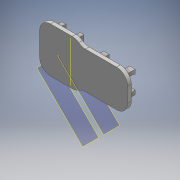
# Autodesk Inventor part: torped2.0
Saved by Autodesk Inventor 2016 (Build 200138000, 138)
## iProperties
Created: 2015-08-25
Part Number: torped2.0
Material: Generic
Document SubType Name: Modeling
Designer: Startic
Density: 1 g/cm^3
Appearance: Default
Author: Startic
Autodesk Inventor part; units mm, degrees
ref_plane "YZ Plane" through (0, 0, 0) normal (1, 0, 0) x (0, 1, 0)
ref_plane "XZ Plane" through (0, 0, 0) normal (0, 1, 0) x (-1, 0, 0)
ref_plane "XY Plane" through (0, 0, 0) normal (0, 0, 1) x (1, 0, 0)
sketch "Sketch1" plane through (0, 0, 0) normal (0, 1, 0) x (-1, 0, 0)
  line L0 (14, 0) -> (-14, 0) projected
  line L1 (0, -17.5) -> (0, 17.5) projected
  line L2 (10, 12.5) -> (-10, 12.5)
  line L3 (-10, 12.5) -> (-10, -12.5)
  line L4 (-10, -12.5) -> (10, -12.5)
  line L5 (10, -12.5) -> (10, 12.5)
  dimension "d0" = 25
  dimension "d1" = 20
  constraints: 8 end point, 2 parallel, 2 symmetric about line, 1 horizontal, 1 perpendicular
  measures "d0" distance of L4.end L2.start
  measures "d1" distance of L3.end L4.end
extrude "Extrusion1" add sketch "Sketch1" along normal blind 2
sketch "Sketch2" plane through (0, 2, 0) normal (0, 1, 0) x (1, 0, 0)
  line L0 (-10, -12.5) -> (10, -12.5) projected
  line L1 (10, -12.5) -> (10, 12.5) projected
  line L2 (10, 12.5) -> (-10, 12.5) projected
  line L3 (-10, 12.5) -> (-10, -12.5) projected
  line L4 (-14, 0) -> (14, 0) projected
  line L5 (0, 17.5) -> (0, -17.5) projected
  line L6 (-6, -8.5) -> (-4, -8.5)
  line L7 (-4, -8.5) -> (-4, -5.5)
  line L8 (-4, -5.5) -> (-6, -5.5)
  line L9 (-6, -5.5) -> (-6, -8.5)
  line L10 (-4.05, 11.55) -> (4.05, 11.55)
  line L11 (4.05, 11.55) -> (4.05, -11.55)
  line L12 (4.05, -11.55) -> (-4.05, -11.55)
  line L13 (-4.05, -11.55) -> (-4.05, 11.55)
  line L14 (-6, 8.5) -> (-6, 5.5)
  line L15 (-4, 8.5) -> (-6, 8.5)
  line L16 (-4, 5.5) -> (-4, 8.5)
  line L17 (-6, 5.5) -> (-4, 5.5)
  line L18 (4, -5.5) -> (4, -8.5)
  line L19 (6, -5.5) -> (4, -5.5)
  line L20 (6, -8.5) -> (6, -5.5)
  line L21 (4, -8.5) -> (6, -8.5)
  line L22 (4, 8.5) -> (4, 5.5)
  line L23 (6, 8.5) -> (4, 8.5)
  line L24 (6, 5.5) -> (6, 8.5)
  line L25 (4, 5.5) -> (6, 5.5)
  dimension "d4" = 8.1
  dimension "d5" = 23.1
  dimension "d6" = 4
  dimension "d7" = 4
  dimension "d8" = 3
  dimension "d9" = 2
  dimension "d12" = 14
  dimension "d15" = 10
  constraints: 40 end point, 4 parallel, 3 horizontal, 2 collinear, 2 perpendicular, 2 symmetric about line, 1 vertical, 22 other
  measures "d4" distance of L11.end L12.end
  measures "d5" distance of L10.end L11.end
  measures "d6" distance between parallel lines of L3 L9
  measures "d7" distance from line of L0.start L6
  measures "d8" distance of L8.end L6.start
  measures "d9" distance of L7.end L8.end
  measures "d12" distance of L8.end L14.start
  measures "d15" distance of L8.end L18.start
extrude "Extrusion2" add sketch "Sketch2" along normal blind 6 contours L13 L6 L9 L8 | L8 L7 L6 L13 | L17 L14 L15 L13 | L13 L15 L16 L17 | L21 L18 L19 L11 | L11 L19 L20 L21 | L25 L22 L23 L11 | L11 L23 L24 L25
sketch "Sketch3" plane through (-6, 2, 8.5) normal (0, 0, 1) x (1, 0, 0)
  line L0 (0, 6) -> (2, 6) projected
  line L1 (2, 0) -> (2, 6) projected
  arc A0 (2.3702, 6) -> (2, 4.2705) centre (6.2252, 4.2705) ccw
  circle A1 centre (6, 4.15) radius 4
  line L2 (-4, 0) -> (16, 0) projected
  line L3 (2, 6) -> (2.3702, 6)
  line L4 (2, 6) -> (2, 4.15)
  line L5 (2, 0) -> (2, 6) projected
  line L6 (6, -4.03) -> (6, 10.18) projected
  line L7 (10, 0) -> (10, 6)
  arc A2 (10, 4.2705) -> (9.6298, 6) centre (5.7748, 4.2705) ccw
  line L8 (10, 6) -> (9.6298, 6)
  dimension "d20" = 4.15
  constraints: 8 end point, 5 symmetric about line, 4 point on circle, 3 point on line, 2 centre point, 1 horizontal, 1 horizontal alignment, 1 tangent, 3 other
  measures "d20" distance from line of point (6, 4.15) L2
extrude "Extrusion4" add sketch "Sketch3" against normal up to surface (3 mm away) from surface at 0 contours L1 L3 A0 | A2 L8 L7
pattern_linear "Rectangular Pattern2" count 2 spacing 14 along (0, 0, -1) of "Extrusion4"
ref_plane "Work Plane2" through (1.3137, 0, 23.8137) normal (-0.7071068, 0, -0.7071068) x (0, -1, 0)
ref_plane "Work Plane1" through (-10, 0, 12.5) normal (-0.7071068, 0, -0.7071068) x (0, -1, 0)
mirror "Mirror1" about plane through (1.3137, 0, 23.8137) normal (-0.7071068, 0, -0.7071068) of "Extrusion1", "Extrusion2", "Extrusion4", "Rectangular Pattern2"
ref_plane "Work Plane3" through (6.6274, 0, 15.1274) normal (-1, 0, 0) x (0, 0, 1)
mirror "Mirror2" about plane through (-10, 0, 12.5) normal (0, 0, 1) of "Extrusion1", "Extrusion2", "Extrusion4", "Rectangular Pattern2"
sketch "Sketch5" plane through (12.6274, 0, 15.1274) normal (0, -1, 0) x (1, 0, 0)
  line L0 (0, 0) -> (25, 0) projected
  line L1 (0, 0) -> (-3, 0)
  line L2 (-3, 0) -> (-3, 20)
  line L3 (-3, 20) -> (0, 20)
  line L4 (0, 20) -> (0, 0)
  constraints: 8 end point, 2 parallel, 1 horizontal, 1 perpendicular
extrude "Extrusion5" add sketch "Sketch5" against normal up to surface (2 mm away)
sketch "Sketch6" plane through (0, 0, 0) normal (0, -1, 0) x (1, 0, 0)
  line L0 (-10, -12.5) -> (-10, 37.5) projected
  line L1 (10, -12.5) -> (-10, -12.5)
  line L2 (-10, -12.5) -> (-10, 13)
  line L3 (-10, 13) -> (10, 13)
  line L4 (10, 13) -> (10, -12.5)
  constraints: 8 end point, 2 parallel, 1 horizontal, 1 perpendicular, 1 point on line
extrude "Extrusion6" cut sketch "Sketch6" against normal through all
fillet "Fillet6" radius 2 21 edges at (33.6274, 2, 30.1274) (33.6274, 2, 20.1274) (32.1274, 2, 19.1274) (30.6274, 2, 30.1274) (30.6274, 2, 20.1274) (32.1274, 2, 31.1274) (18.1274, 2, 31.1274) (19.6274, 2, 30.1274) (16.6274, 2, 30.1274) (5, 2, 33.5) (-5, 2, 33.5) (-6, 2, 32) (-6, 2, 18) (16.6274, 2, 20.1274) (5, 2, 30.5) (18.1274, 2, 19.1274) (5, 2, 16.5) (-5, 2, 16.5) (6, 2, 32) (6, 2, 18) (19.6274, 2, 20.1274)
fillet "Fillet7" radius 6 8 edges at (37.6274, 1, 15.1274) (10, 1, 15.1274) (10, 1, 13) (37.6274, 1, 35.1274) (10, 1, 35.1274) (10, 1, 37.5) (-10, 1, 37.5) (-10, 1, 13)
body "Solid1"
